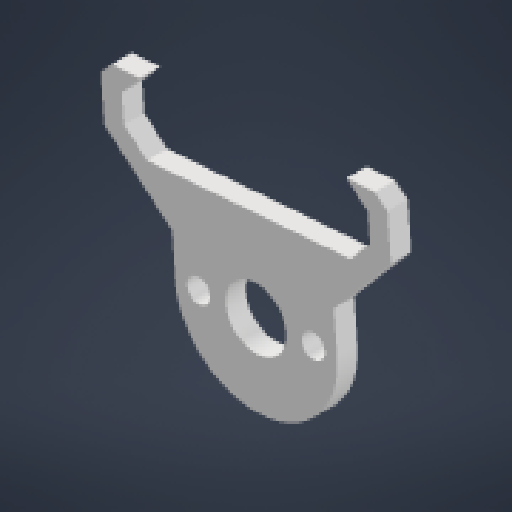
# Autodesk Inventor part: Elevation_mount
Saved by Autodesk Inventor 2023.4 (Build 274418000, 418)
## iProperties
Created: 2025-10-08
Part Number: Elevation_mount
Material: Generic
Document SubType Name: Modeling
Designer: Malthe Sennels
Density: 1 g/cm^3
Appearance: Default
Author: Malthe Sennels
Autodesk Inventor part; units mm, degrees
ref_plane "YZ Plane" through (0, 0, 0) normal (1, 0, 0) x (0, 1, 0)
ref_plane "XZ Plane" through (0, 0, 0) normal (0, 1, 0) x (-1, 0, 0)
ref_plane "XY Plane" through (0, 0, 0) normal (0, 0, 1) x (1, 0, 0)
sketch "Sketch1" plane through (0, 0, 0) normal (0, 0, 1) x (1, 0, 0)
  line L0 (13.859678, 14.743814) -> (-16.04324, 12.332282)
  line L1 (-19.274685, 15.081421) -> (-16.04324, 12.332282)
  line L2 (-19.274685, 15.081421) -> (-19.435453, 17.074949)
  line L3 (-19.435453, 17.074949) -> (-19.584165, 18.918962)
  line L4 (16.608817, 17.975258) -> (13.859678, 14.743814)
  line L5 (16.608817, 17.975258) -> (16.448048, 19.968786)
  line L6 (16.448048, 19.968786) -> (16.299337, 21.8128)
  circle A0 centre (0, 0) radius 3.5
  circle A1 centre (0, 0) radius 12
  line L7 (0, 0) -> (-1.091781, 13.538048)
  line L8 (0, 0) -> (8.472493, 0.683267)
  circle A2 centre (8.472493, 0.683267) radius 1.75
  circle A3 centre (-8.472493, -0.683267) radius 1.75
  line L9 (-16.835026, 22.150407) -> (-19.584165, 18.918962)
  line L10 (13.067892, 24.561938) -> (16.299337, 21.8128)
  line L11 (-17.116953, 22.127671) -> (-19.790177, 18.98546)
  line L12 (-19.790177, 18.98546) -> (-19.634806, 17.058872)
  line L13 (-19.634806, 17.058872) -> (-19.467378, 14.982769)
  line L14 (-19.467378, 14.982769) -> (-16.109737, 12.12627)
  line L15 (-16.109737, 12.12627) -> (13.95833, 14.55112)
  line L16 (13.95833, 14.55112) -> (16.814829, 17.908761)
  line L17 (16.814829, 17.908761) -> (16.647401, 19.984863)
  line L18 (16.647401, 19.984863) -> (16.492031, 21.911451)
  line L19 (16.492031, 21.911451) -> (13.34982, 24.584674)
  line L20 (-21.345865, 21.786629) -> (-22.880357, 19.982926)
  line L21 (-22.880357, 19.982926) -> (-22.625098, 16.817719)
  line L22 (-22.625098, 16.817719) -> (-22.357781, 13.502997)
  line L23 (-22.357781, 13.502997) -> (-17.107204, 9.036089)
  line L24 (-17.107204, 9.036089) -> (15.438103, 11.660717)
  line L25 (15.438103, 11.660717) -> (19.90501, 16.911294)
  line L26 (19.90501, 16.911294) -> (19.637693, 20.226016)
  line L27 (19.637693, 20.226016) -> (19.382434, 23.391224)
  line L28 (19.382434, 23.391224) -> (17.578731, 24.925717)
  line L29 (-12.795718, 9.383791) -> (-11.961167, -0.964613)
  line L30 (11.126617, 11.313016) -> (11.961167, 0.964613)
  line L31 (-17.107204, 9.036089) -> (-12.448017, 5.072305)
  line L32 (15.438103, 11.660717) -> (11.474318, 7.00153)
  circle A4 centre (0, 0) radius 3.5
  circle A5 centre (0, 0) radius 4.5
  line L33 (-17.116953, 22.127671) -> (-21.345865, 21.786629)
  line L34 (13.34982, 24.584674) -> (17.578731, 24.925717)
  point P0 (0, 0)
  point P1 (11.961167, 0.964613)
  dimension "d0" = 3.5
  dimension "d1" = 8.5
  dimension "d4" = 360
  dimension "d6" = 0.2
  dimension "d7" = 3
  dimension "d8" = 1
  constraints: 54 end point, 4 point on line, 3 centre point, 3 perpendicular, 3 symmetric about line, 2 coincident, 2 parallel, 1 collinear, 1 midpoint, 26 other
  measures "d0" diameter of A2
  measures "d1" distance of point (0, 0) L8.end
  measures "d6" distance between parallel lines of L9 L11
  measures "d7" distance between parallel lines of L20 L11
  measures "d8" radial gap between concentric circles of A0 A5
extrude "Extrusion1" add sketch "Sketch1" along normal blind 3
sketch "Sketch2" plane through (0, 0, 0) normal (0, 0, -1) x (-1, 0, 0)
  circle A0 centre (0, 0) radius 12
  line L0 (-11.961167, 0.964613) -> (-11.474318, 7.00153)
  arc A1 (-11.961167, 0.964613) -> (11.961167, -0.964613) centre (0, 0) ccw
  line L1 (12.448017, 5.072305) -> (11.961167, -0.964613)
  line L2 (22.357781, 13.502997) -> (12.448017, 5.072305)
  line L3 (22.880357, 19.982926) -> (22.357781, 13.502997)
  line L4 (21.345865, 21.786629) -> (22.880357, 19.982926)
  line L5 (17.116953, 22.127671) -> (21.345865, 21.786629)
  line L6 (19.790177, 18.98546) -> (17.116953, 22.127671)
  line L7 (19.467378, 14.982769) -> (19.790177, 18.98546)
  line L8 (16.109737, 12.12627) -> (19.467378, 14.982769)
  line L9 (-13.95833, 14.55112) -> (16.109737, 12.12627)
  line L10 (-16.814829, 17.908761) -> (-13.95833, 14.55112)
  line L11 (-16.492031, 21.911451) -> (-16.814829, 17.908761)
  line L12 (-13.34982, 24.584674) -> (-16.492031, 21.911451)
  line L13 (-17.578731, 24.925717) -> (-13.34982, 24.584674)
  line L14 (-19.382434, 23.391224) -> (-17.578731, 24.925717)
  line L15 (-19.90501, 16.911294) -> (-19.382434, 23.391224)
  line L16 (-11.474318, 7.00153) -> (-19.90501, 16.911294)
  circle A2 centre (-8.472493, 0.683267) radius 1.75
  circle A3 centre (8.472493, -0.683267) radius 1.75
  circle A4 centre (0, 0) radius 4.5
  point P0 (0, 0)
  point P1 (11.961167, -0.964613)
extrude "Extrusion2" add sketch "Sketch2" along normal blind 30 contours A0 L0 L16 L15 L14 L13 L12 L11 L10 L9 L8 L7 L6 L5 L4 L3 L2 L1
fillet "Fillet1" radius 0.5 2 edges at (11.9612, 0.9646, -15) (-11.9612, -0.9646, -15)
sketch "Sketch3" plane through (13.34982, 24.584674, 3) normal (-0.0803844, 0.9967639, 0) x (0.9967639, 0.0803844, 0)
  line L0 (9.913898, 10) -> (-40.53242, 10)
  line L1 (-40.53242, 10) -> (-40.53242, 20)
  line L2 (-40.53242, 20) -> (9.913898, 20)
  line L3 (9.913898, 20) -> (9.913898, 10)
  line L4 (-34.808326, 0) -> (-36.482843, 0)
  point P0 (-15.282843, 3)
  dimension "d14" = 10
  dimension "d15" = 10
  constraints: 8 end point, 2 parallel, 1 horizontal, 1 perpendicular
  measures "d14" distance of L0.end L1.end
  measures "d15" distance between parallel lines of L4 L0
extrude "Extrusion3" cut sketch "Sketch3" against normal up to surface (10.05 mm away)
chamfer "Chamfer1" distance 2 angle 45 2 edges at (18.1872, 14.8922, -12) (-20.3386, 11.7852, -12)
sketch "Sketch4" plane through (0, 0, -30) normal (0, 0, -1) x (-1, 0, 0)
  circle A0 centre (0, 0) radius 12
  circle A1 centre (0, 0) radius 15
  line L0 (-14.951459, 1.205766) -> (-14.223457, 10.232975)
  line L1 (-11.474318, 7.00153) -> (-19.90501, 16.911294)
  line L2 (16.109737, 12.12627) -> (-13.95833, 14.55112)
  line L3 (0, 0) -> (1.075704, 13.338695)
  line L4 (14.951459, -1.205766) -> (15.679462, 7.821443)
  circle A2 centre (0, 0) radius 12.2
  line L5 (12.448017, 5.072305) -> (22.357781, 13.502997)
  point P0 (0, 0)
  point P1 (-5.67895, 13.883426)
  point P2 (-12.531386, 8.24405)
  point P3 (13.690536, 6.129373)
  point P4 (7.830357, 12.793964)
  dimension "d21" = 3
  dimension "d22" = 0.2
  constraints: 6 end point, 2 symmetric about line, 1 centre point, 1 midpoint, 1 perpendicular, 1 point on line, 4 other
  measures "d22" radial gap between concentric circles of A0 A2
extrude "Extrusion4" add sketch "Sketch4" against normal blind 5 contours A1 L2 | L0 L1 A1 | A1 L5 L4 picked at (4.282071, 12.559626)
body "Solid1"
